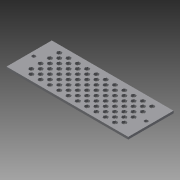
# Autodesk Inventor part: side
Saved by Autodesk Inventor 2013 SP1 (Build 170176100, 176)
## iProperties
Created: 2019-01-15
Part Number: side
Material: Типовые
Document SubType Name: Modeling
Designer: jhcjhguw
Density: 1 g/cm^3
Author: jhcjhguw
Autodesk Inventor part; units mm, degrees
ref_plane "YZ Plane" through (0, 0, 0) normal (1, 0, 0) x (0, 1, 0)
ref_plane "XZ Plane" through (0, 0, 0) normal (0, 1, 0) x (-1, 0, 0)
ref_plane "XY Plane" through (0, 0, 0) normal (0, 0, 1) x (1, 0, 0)
sketch "Эскиз1" plane through (0, 0, 0) normal (0, 0, 1) x (1, 0, 0)
  line L0 (0, 0) -> (104.8, 0)
  line L1 (104.8, 0) -> (104.8, 39)
  line L2 (104.8, 39) -> (0, 39)
  line L3 (0, 39) -> (0, 0)
  dimension "d0" = 104.8
  dimension "d1" = 39
  constraints: 8 end point, 2 parallel, 1 horizontal, 1 perpendicular
  measures "d0" distance of L2.end L1.end
  measures "d1" distance of L1.end L0.end
extrude "Выдавливание1" add sketch "Эскиз1" along normal blind 2
sketch "Эскиз2" plane through (0, 0, 2) normal (0, 0, 1) x (1, 0, 0)
  line L0 (104.8, 39) -> (0, 39) projected
  line L1 (0, 39) -> (0, 0) projected
  line L2 (13.4, 34.7321) -> (14.4, 33)
  line L3 (14.4, 33) -> (13.4, 31.2679)
  line L4 (13.4, 31.2679) -> (11.4, 31.2679)
  line L5 (11.4, 31.2679) -> (10.4, 33)
  line L6 (10.4, 33) -> (11.4, 34.7321)
  line L7 (11.4, 34.7321) -> (13.4, 34.7321)
  point P0 (12.4, 33)
  point P1 (12.4, 34.7321)
  dimension "d4" = 2
  dimension "d6" = 6
  dimension "d7" = 12.4
  constraints: 12 end point, 1 horizontal, 1 midpoint, 13 other
  measures "d4" distance of L3.end L4.end
  measures "d6" distance from line of L0 point (12.4, 33)
  measures "d7" distance from line of L1 point (12.4, 33)
extrude "Выдавливание2" cut sketch "Эскиз2" against normal blind 2
pattern_linear "Прямоуг.массив1" count 11 spacing 8 along (1, 0, 0) count 4 spacing 8 along (0, -1, 0) of "Выдавливание2"
sketch "Эскиз3" plane through (0, 0, 2) normal (0, 0, 1) x (1, 0, 0)
  line L0 (104.8, 39) -> (0, 39) projected
  line L1 (0, 39) -> (0, 0) projected
  line L2 (17.4, 30.7321) -> (18.4, 29)
  line L3 (18.4, 29) -> (17.4, 27.2679)
  line L4 (17.4, 27.2679) -> (15.4, 27.2679)
  line L5 (15.4, 27.2679) -> (14.4, 29)
  line L6 (14.4, 29) -> (15.4, 30.7321)
  line L7 (15.4, 30.7321) -> (17.4, 30.7321)
  point P0 (16.4, 29)
  dimension "d16" = 2
  dimension "d17" = 10
  dimension "d18" = 16.4
  constraints: 12 end point, 1 horizontal, 13 other
  measures "d16" distance of L3.end L4.end
  measures "d17" distance from line of L0 point (16.4, 29)
  measures "d18" distance from line of L1 point (16.4, 29)
extrude "Выдавливание3" cut sketch "Эскиз3" against normal blind 2
pattern_linear "Прямоуг.массив2" count 10 spacing 8 along (1, 0, 0) count 4 spacing 8 along (0, -1, 0) of "Выдавливание3"
sketch "Эскиз4" plane through (0, 0, 2) normal (0, 0, 1) x (1, 0, 0)
  line L0 (0, 0) -> (104.8, 0) projected
  line L1 (104.8, 0) -> (104.8, 39) projected
  line L2 (104.8, 39) -> (0, 39) projected
  line L3 (0, 39) -> (0, 0) projected
  circle A0 centre (4, 19.5) radius 1.5
  circle A1 centre (100.8, 19.5) radius 1.5
  dimension "d27" = 3
  dimension "d28" = 3
  dimension "d29" = 39
  dimension "d30" = 19.5
  dimension "d31" = 19.5
  dimension "d32" = 4
  dimension "d33" = 4
  constraints: 2 centre point
  measures "d27" diameter of A0
  measures "d28" diameter of A1
  measures "d29" distance between parallel lines of L0 L2
  measures "d30" distance from line of A0.centre L0
  measures "d31" distance from line of L0 A1.centre
  measures "d32" distance from line of L3 A0.centre
  measures "d33" distance from line of L1 A1.centre
extrude "Выдавливание4" cut sketch "Эскиз4" against normal blind 2 contours A0 | A1
